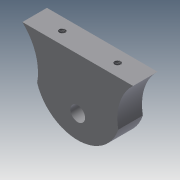
# Autodesk Inventor part: stojan
Saved by Autodesk Inventor 2013 (Build 170138000, 138)
## iProperties
Created: 2013-05-11
Part Number: stojan
Material: Generic
Document SubType Name: Modeling
Designer: idle-rug
Density: 1 g/cm^3
Author: idle-rug
Autodesk Inventor part; units mm, degrees
ref_plane "YZ Plane" through (0, 0, 0) normal (1, 0, 0) x (0, 1, 0)
ref_plane "XZ Plane" through (0, 0, 0) normal (0, 1, 0) x (-1, 0, 0)
ref_plane "XY Plane" through (0, 0, 0) normal (0, 0, 1) x (1, 0, 0)
sketch "Sketch1" plane through (0, 0, 0) normal (0, 1, 0) x (-1, 0, 0)
  line L0 (-22.5, 13) -> (22.5, 13)
  circle A0 centre (0, 0) radius 3
  arc A1 (-16.4878, -5.3902) -> (16.4878, -5.3902) centre (0, 0) ccw
  arc A2 (22.5, 13) -> (16.4878, -5.3902) centre (36.132, -1.6345) ccw
  arc A3 (-16.4878, -5.3902) -> (-22.5, 13) centre (-36.132, -1.6345) ccw
  arc A4 (-16.4878, -5.3902) -> (16.4878, -5.3902) centre (0, 0) ccw
  arc A5 (22.5, 13) -> (16.4878, -5.3902) centre (36.132, -1.6345) ccw
  arc A6 (-16.4878, -5.3902) -> (-22.5, 13) centre (-36.132, -1.6345) ccw
  line L1 (22.5, 13) -> (-22.5, 13)
  dimension "d0" = 45
  dimension "d4" = 6
  dimension "d5" = 20
  dimension "d6" = 20
  constraints: 12 point on circle, 7 centre point, 4 end point, 3 concentric, 1 coincident, 1 collinear
  measures "d0" distance of L0.start L0.end
  measures "d4" diameter of A0
  measures "d5" radius of A2
  measures "d6" radius of A3
extrude "Extrusion1" add sketch "Sketch1" along normal blind 10
sketch "Sketch2" plane through (-22.5, 0, 13) normal (0, 0, 1) x (1, 0, 0)
  circle A0 centre (11.25, 5) radius 1.5
  circle A1 centre (33.75, 5) radius 1.5
  point P0 (22.5, 0)
  dimension "d10" = 3
  dimension "d11" = 3
  constraints: 2 centre point
  measures "d10" diameter of A0
  measures "d11" diameter of A1
hole "Hole1" at (11.25, 5, 13) at (-11.25, 5, 13) direction (0, 0, -1) diameter 2.459 depth 8 tip angle 118 thread size "M3x0.5" class "6H" standard "ISO Metric profile"
sketch "Sketch3" plane through (0, 0, 0) normal (0, -1, 0) x (1, 0, 0)
  circle A0 centre (0, 0) radius 3 projected
extrude "Extrusion2" add sketch "Sketch3" against normal blind 10
sketch "Sketch4" plane through (0, 0, 0) normal (0, -1, 0) x (1, 0, 0)
  line L0 (-22.5, 13) -> (22.5, 13) projected
  line L1 (0, 13) -> (0, -8)
  circle A0 centre (0, -8) radius 3
  dimension "d21" = 21
  dimension "d22" = 6
  constraints: 2 end point, 1 centre point, 1 coincident, 1 midpoint, 1 perpendicular
  measures "d21" distance of L1.start L1.end
  measures "d22" diameter of A0
extrude "Extrusion3" cut sketch "Sketch4" against normal blind 10
body "Solid1"
